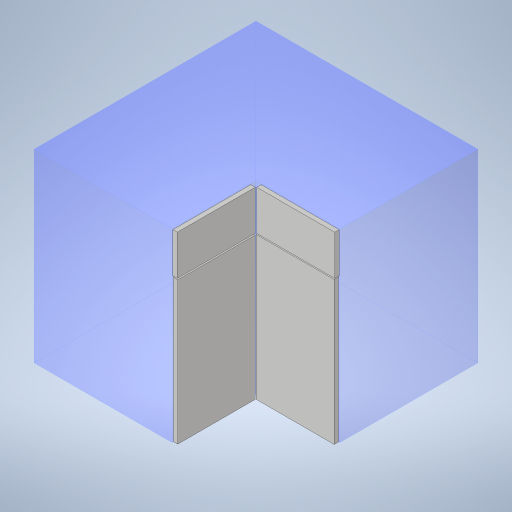
# Autodesk Inventor part: Placed 90 d corner cabinet door
Saved by Autodesk Inventor 2024 (Build 280153000, 153)
## iProperties
Created: 2017-01-30
Part Number: Placed 90 d corner cabinet door
Material: Generic
Document SubType Name: Modeling
Designer: SvetlanaB
Density: 1 g/cm^3
Appearance: Default
Author: SvetlanaB
Autodesk Inventor part; units mm, degrees
ref_plane "YZ Plane" through (0, 0, 0) normal (1, 0, 0) x (0, 1, 0)
ref_plane "XZ Plane" through (0, 0, 0) normal (0, 1, 0) x (-1, 0, 0)
sketch "Sketch1" plane through (0, 0, 0) normal (0, 0, 1) x (1, 0, 0)
  line L0 (-450, 450) -> (450, 450)
  line L1 (450, 450) -> (450, -450)
  line L2 (450, -450) -> (-450, -450)
  line L3 (-450, -450) -> (-450, 450)
  line L4 (-450, 450) -> (450, -450) construction
  line L5 (450, 450) -> (-450, -450) construction
  point P0 (0, 0)
  dimension "Width" = 900
  dimension "Depth" = 900
  constraints: 12 end point, 2 midpoint, 2 parallel, 1 horizontal, 1 perpendicular
  measures "Width" distance of L1.end L2.end
  measures "Depth" distance between parallel lines of L2 L0
extrude "Extrusion1" add sketch "Sketch1" along normal blind 850
move faces "Move1" translate (0, 0, 100) faces at (-150, -150, 0)
sketch "Sketch2" plane through (0, 0, 850) normal (0, 0, 1) x (1, 0, 0)
  line L0 (450, 450) -> (-450, 450) projected
  line L1 (-450, 450) -> (-450, -450) projected
  line L2 (-450, -450) -> (450, -450) projected
  line L3 (450, -450) -> (450, 450) projected
  line L4 (450, -450) -> (450, 450) projected
  line L5 (450, -110) -> (110, -450)
  line L6 (-450, -450) -> (450, -450) projected
  point P0 (0, 0)
  dimension "d4" = 560
  dimension "d5" = 560
  constraints: 2 end point, 2 point on line
  measures "d4" distance from line of L0 L5.start
  measures "d5" distance from line of L1 L5.end
extrude "Extrusion2" cut sketch "Sketch2" against normal up to surface (850 mm away) contours L3 L2 L5
sketch "Sketch6" plane through (0, 0, 850) normal (0, 0, 1) x (1, 0, 0)
  line L0 (110, -450) -> (450, -110) projected
  line L1 (450, -110) -> (450, 450) projected
  line L2 (450, 450) -> (-450, 450) projected
  line L3 (-450, 450) -> (-450, -450) projected
  line L4 (-450, -450) -> (110, -450) projected
  line L5 (110, -450) -> (110, -110)
  line L6 (110, -110) -> (450, -110)
  point P0 (0, 0)
  constraints: 4 end point, 1 perpendicular
extrude "Extrusion7" cut sketch "Sketch6" against normal up to surface (750 mm away) contours L5 L6 L0
ref_plane "Work Plane1" through (0, 0, 684) normal (0, 0, 1) x (1, 0, 0)
sketch "Sketch7" plane through (110, -110, 850) normal (0, -1, 0) x (1, 0, 0)
  line L0 (340, -750) -> (0, -750) construction
  line L1 (340, 0) -> (340, -750) construction
  line L2 (0, 0) -> (340, 0) construction
  line L3 (0, 0) -> (0, -750) construction
  line L4 (-740, -166) -> (520, -166) construction
  line L5 (21, -4) -> (337, -4)
  line L6 (337, -4) -> (337, -166)
  line L7 (337, -166) -> (21, -166)
  line L8 (21, -166) -> (21, -4)
  point P0 (-110, -850)
  dimension "d33" = 3
  dimension "d34" = 21
  dimension "d35" = 4
  constraints: 8 end point, 2 parallel, 1 collinear, 1 horizontal, 1 perpendicular
  measures "d33" distance between parallel lines of L1 L6
  measures "d34" distance between parallel lines of L3 L8
  measures "d35" distance between parallel lines of L2 L5
extrude "Extrusion8" add sketch "Sketch7" along normal blind 18 separate body
sketch "Sketch8" plane through (110, -110, 850) normal (0, -1, 0) x (1, 0, 0)
  line L0 (340, -750) -> (0, -750) construction
  line L1 (340, 0) -> (340, -750) construction
  line L2 (0, 0) -> (340, 0) construction
  line L3 (0, 0) -> (0, -750) construction
  line L4 (337, -4) -> (21, -4) construction
  line L5 (21, -4) -> (21, -166) construction
  line L6 (21, -166) -> (337, -166) construction
  line L7 (337, -166) -> (337, -4) construction
  line L8 (21, -169) -> (337, -169)
  line L9 (337, -169) -> (337, -748)
  line L10 (337, -748) -> (21, -748)
  line L11 (21, -748) -> (21, -169)
  point P0 (-110, -850)
  dimension "d38" = 2
  dimension "d39" = 3
  dimension "d40" = 21
  dimension "d41" = 3
  constraints: 8 end point, 2 parallel, 1 horizontal, 1 perpendicular
  measures "d38" distance between parallel lines of L0 L10
  measures "d39" distance between parallel lines of L1 L9
  measures "d40" distance between parallel lines of L3 L11
  measures "d41" distance between parallel lines of L6 L8
extrude "Extrusion9" add sketch "Sketch8" along normal blind 18 separate body
move or copy body "Move4" bodies to move or copy 3 copy no translate (0, -2, 0)
sketch "Sketch9" plane through (110, -450, 850) normal (1, 0, 0) x (0, 0, -1)
  line L0 (750, 340) -> (750, 0) construction
  line L1 (0, 340) -> (750, 340) construction
  line L2 (0, 0) -> (0, 340) construction
  line L3 (750, 0) -> (0, 0) construction
  line L4 (166, -180) -> (166, 1080) construction
  line L5 (4, 3) -> (166, 3)
  line L6 (166, 3) -> (166, 319)
  line L7 (166, 319) -> (4, 319)
  line L8 (4, 319) -> (4, 3)
  line L9 (4, 340) -> (166, 340) projected
  line L10 (4, 340) -> (4, 322) projected
  line L11 (166, 322) -> (4, 322) projected
  line L12 (166, 340) -> (166, 322) projected
  point P0 (850, 450)
  dimension "d53" = 3
  dimension "d54" = 4
  dimension "d55" = 3
  constraints: 8 end point, 2 parallel, 1 collinear, 1 horizontal, 1 perpendicular
  measures "d53" distance between parallel lines of L3 L5
  measures "d54" distance between parallel lines of L2 L8
  measures "d55" distance between parallel lines of L11 L7
extrude "Extrusion10" add sketch "Sketch9" along normal blind 18 separate body contours L8 L7 L6 L5
sketch "Sketch10" plane through (110, -450, 850) normal (1, 0, 0) x (0, 0, -1)
  line L0 (750, 340) -> (750, 0) construction
  line L1 (0, 340) -> (750, 340) construction
  line L2 (0, 0) -> (0, 340) construction
  line L3 (750, 0) -> (0, 0) construction
  line L4 (4, 3) -> (166, 3) construction
  line L5 (166, 3) -> (166, 319) construction
  line L6 (166, 319) -> (4, 319) construction
  line L7 (4, 319) -> (4, 3) construction
  line L8 (170, 3) -> (747, 3)
  line L9 (747, 3) -> (747, 317)
  line L10 (747, 317) -> (170, 317)
  line L11 (170, 317) -> (170, 3)
  line L12 (169, 338) -> (748, 338) projected
  line L13 (169, 338) -> (169, 320) projected
  line L14 (748, 320) -> (169, 320) projected
  line L15 (748, 338) -> (748, 320) projected
  point P0 (850, 450)
  dimension "d58" = 3
  dimension "d59" = 3
  dimension "d60" = 3
  dimension "d61" = 4
  constraints: 8 end point, 2 parallel, 1 horizontal, 1 perpendicular
  measures "d58" distance between parallel lines of L0 L9
  measures "d59" distance between parallel lines of L14 L10
  measures "d60" distance between parallel lines of L3 L8
  measures "d61" distance between parallel lines of L5 L11
extrude "Extrusion11" add sketch "Sketch10" along normal blind 18 separate body contours L11 L10 L9 L8
move or copy body "Move5" bodies to move or copy 5 copy no translate (2, 0, 0)
equation "\"d36\" = Panel_thickness"
equation "\"d42\" = Panel_thickness"
equation "\"d56\" = Panel_thickness"
equation "\"d62\" = Panel_thickness"
equation "\"Panel_thickness\" = 18"
